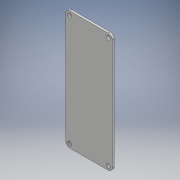
# Autodesk Inventor part: Power Supply
Saved by Autodesk Inventor 2018 (Build 220112000, 112)
## iProperties
Created: 2018-09-04
Part Number: Power Supply
Material: Generic
Document SubType Name: Modeling
Designer: matth
Density: 1 g/cm^3
Appearance: Default
Author: matth
Autodesk Inventor part; units mm, degrees
ref_plane "YZ Plane" through (0, 0, 0) normal (1, 0, 0) x (0, 1, 0)
ref_plane "XZ Plane" through (0, 0, 0) normal (0, 1, 0) x (-1, 0, 0)
ref_plane "XY Plane" through (0, 0, 0) normal (0, 0, 1) x (1, 0, 0)
sketch "Sketch1" plane through (0, 0, 0) normal (0, 1, 0) x (-1, 0, 0)
  line L0 (0, 0) -> (29.141, 0)
  line L1 (29.141, 83.82) -> (0, 83.82)
  line L2 (0, 83.82) -> (0, 86.82)
  line L3 (0, 86.82) -> (-3, 86.82)
  line L4 (-3, 86.82) -> (32.141, 86.82)
  line L5 (32.141, 86.82) -> (32.141, -3)
  line L6 (32.141, -3) -> (-3, -3)
  line L7 (-3, -3) -> (-3, 86.82)
  circle A0 centre (0, 83.82) radius 1.5
  circle A1 centre (29.141, 83.82) radius 1.5
  circle A2 centre (0, 0) radius 1.5
  circle A3 centre (29.141, 0) radius 1.5
  dimension "d0" = 29.141
  dimension "d1" = 83.82
  dimension "d2" = 3
  dimension "d3" = 3
  dimension "d4" = 35.141
  dimension "d5" = 89.82
  dimension "d6" = 3
  dimension "d7" = 3
  dimension "d8" = 3
  dimension "d9" = 3
  constraints: 16 end point, 4 centre point, 4 coincident, 3 parallel, 2 horizontal, 2 perpendicular, 1 vertical
  measures "d0" distance of L1.end L1.start
  measures "d1" distance of L1.start L0.end
  measures "d2" distance of L1.end L2.end
  measures "d3" distance of L2.end L3.end
  measures "d4" distance of L5.end L6.end
  measures "d5" distance of L4.end L5.end
  measures "d6" diameter of A0
  measures "d7" diameter of A1
  measures "d8" diameter of A2
  measures "d9" diameter of A3
extrude "Extrusion1" add sketch "Sketch1" along normal blind 1.5
fillet "Fillet1" radius 3 4 edges at (-32.141, 0.75, 86.82) (3, 0.75, 86.82) (3, 0.75, -3) (-32.141, 0.75, -3)
body "Solid1"
